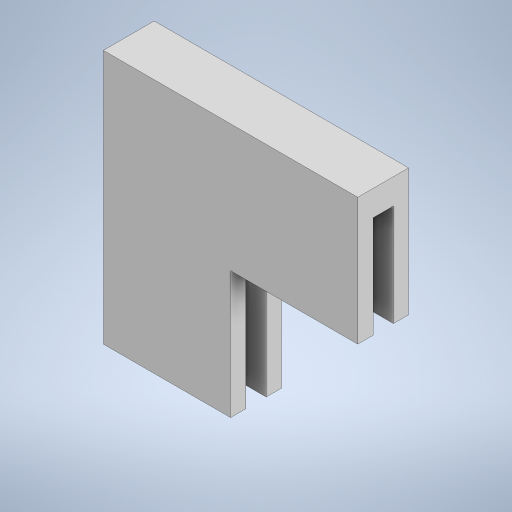
# Autodesk Inventor part: Eckenbohren
Saved by Autodesk Inventor 2024 (Build 280153000, 153)
## iProperties
Created: 2025-02-21
Part Number: Eckenbohren
Material: Generisch
Document SubType Name: Sheet Metal
Designer: Carla
Density: 1 g/cm^3
Sheet Metal Rule: Standard_mm
Appearance: Vorgabe
Author: Carla
Autodesk Inventor part; units mm, degrees
ref_plane "YZ Plane" through (0, 0, 0) normal (1, 0, 0) x (0, 1, 0)
ref_plane "XZ Plane" through (0, 0, 0) normal (0, 1, 0) x (-1, 0, 0)
ref_plane "XY Plane" through (0, 0, 0) normal (0, 0, 1) x (1, 0, 0)
sketch "Skizze1" plane through (0, 0, 0) normal (0, 1, 0) x (-1, 0, 0)
  line L0 (0, 0) -> (-50, 0)
  line L1 (-50, 0) -> (-50, 25)
  line L2 (-50, 25) -> (0, 25)
  line L3 (0, 25) -> (0, 0)
  line L4 (0, 0) -> (-25, 0)
  line L5 (-25, 0) -> (-25, -25)
  line L6 (-25, -25) -> (0, -25)
  line L7 (0, -25) -> (0, 0)
  dimension "d0" = 50
  dimension "d1" = 25
  dimension "d2" = 25
  dimension "d3" = 25
  constraints: 16 end point, 4 parallel, 2 horizontal, 2 perpendicular
  measures "d0" distance of L1.end L2.end
  measures "d1" distance of L2.end L0.start
  measures "d2" distance of L5.end L6.end
  measures "d3" distance of L6.end L0.start
extrude "Extrusion1" add sketch "Skizze1" along normal blind 10
sketch "Skizze2" plane through (50, 0, 25) normal (1, 0, 0) x (0, 0, -1)
  line L0 (25, 0) -> (25, 10) projected
  line L1 (25, 7) -> (5, 7)
  line L2 (5, 7) -> (5, 3)
  line L3 (5, 3) -> (25, 3)
  line L4 (25, 3) -> (25, 7)
  line L5 (0, 10) -> (25, 10) projected
  line L6 (0, 0) -> (25, 0) projected
  point P0 (12.5, 10)
  dimension "d6" = 3
  dimension "d7" = 3
  dimension "d8" = 20
  constraints: 8 end point, 2 parallel, 1 horizontal, 1 midpoint, 1 perpendicular, 1 point on line
  measures "d6" distance from line of point (12.5, 10) L1
  measures "d7" distance between parallel lines of L6 L3
  measures "d8" distance of L1.start L1.end
extrude "Extrusion2" cut sketch "Skizze2" against normal blind 45
sketch "Skizze3" plane through (25, 0, -25) normal (0, 0, -1) x (-1, 0, 0)
  line L0 (0, 3) -> (20, 3) projected
  line L1 (20, 7) -> (20, 3) projected
  line L2 (0, 3) -> (20, 3)
  line L3 (20, 3) -> (20, 7)
  line L4 (20, 7) -> (0, 7)
  line L5 (0, 7) -> (0, 3)
  point P0 (25, 0)
  constraints: 8 end point, 2 parallel, 1 horizontal, 1 perpendicular
extrude "Extrusion3" cut sketch "Skizze3" against normal blind 45
sketch "Skizze4" plane through (0, 10, 0) normal (0, 1, 0) x (1, 0, 0)
  line L0 (50, -20) -> (5, -20) projected
  line L1 (25, 0) -> (5, 0)
  line L2 (5, 0) -> (5, -20)
  line L3 (5, -20) -> (25, -20)
  line L4 (25, -20) -> (25, 0)
  line L5 (5, -20) -> (35, -20)
  line L6 (35, -20) -> (35, 10)
  line L7 (35, 10) -> (5, 10)
  line L8 (5, 10) -> (5, -20)
  circle A0 centre (20, -5) radius 1.7
  point P0 (0, 0)
  dimension "d13" = 30
  dimension "d14" = 30
  dimension "d15" = 3.4
  constraints: 16 end point, 4 parallel, 2 horizontal, 2 perpendicular, 1 centre point
  measures "d13" distance of L6.end L7.end
  measures "d14" distance of L5.end L6.end
  measures "d15" diameter of A0
extrude "Extrusion4" cut sketch "Skizze4" against normal blind 3 contours A0
equation "\"Biegeradius\" = Stärke"
equation "\"BreiteBiegungsfreistellung\" = Stärke"
equation "\"TiefeBiegungsfreistellung\" = 0.5 * Stärke"
equation "\"GrößeEckenfreistellung\" = 4 * Stärke"
equation "\"MinimalRest\" = 2 * Stärke"
equation "\"Übergangsradius\" = Biegeradius"
equation "\"JacobiRadiusGröße\" = Biegeradius"
equation "\"Abstandsgröße\" = Stärke"
equation "\"Stärke\" = 0.5"
